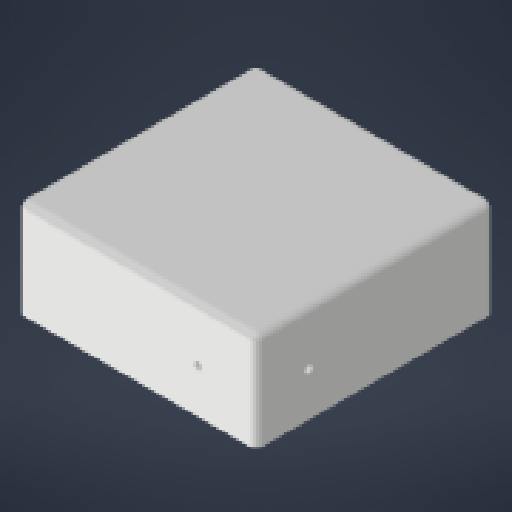
# Autodesk Inventor part: PCB_Housing_02
Saved by Autodesk Inventor 2026.2 (Build 302298000, 298)
## iProperties
Created: 2026-02-05
Part Number: PCB_Housing_02
Material: Generic
Document SubType Name: Modeling
Designer: vckot
Density: 1 g/cm^3
Appearance: Default
Author: vckot
Autodesk Inventor part; units mm, degrees
ref_plane "YZ Plane" through (0, 0, 0) normal (1, 0, 0) x (0, 1, 0)
ref_plane "XZ Plane" through (0, 0, 0) normal (0, 1, 0) x (-1, 0, 0)
ref_plane "XY Plane" through (0, 0, 0) normal (0, 0, 1) x (1, 0, 0)
sketch "Sketch1" plane through (0, 0, 0) normal (0, 1, 0) x (-1, 0, 0)
  line L0 (-85, 85) -> (85, 85)
  line L1 (85, 85) -> (85, -85)
  line L2 (85, -85) -> (-85, -85)
  line L3 (-85, -85) -> (-85, 85)
  line L4 (-85, 85) -> (85, -85) construction
  line L5 (85, 85) -> (-85, -85) construction
  point P0 (0, 0)
  dimension "d0" = 170
  dimension "d1" = 170
  constraints: 12 end point, 2 midpoint, 2 parallel, 1 horizontal, 1 perpendicular
  measures "d0" distance of L0.end L1.end
  measures "d1" distance of L1.end L2.end
extrude "Extrusion1" add sketch "Sketch1" along normal blind 70
fillet "Fillet1" radius 5 8 edges at (0, 70, 85) (85, 70, 0) (-85, 70, 0) (-85, 35, 85) (85, 35, 85) (85, 35, -85) (0, 70, -85) (-85, 35, -85)
shell "Shell1" thickness 4 removed faces 1 at (28.3333, 0, -26.6667)
sketch "Sketch2" plane through (85, 0, 80) normal (1, 0, 0) x (0, 0, -1)
  point P0 (80, 0)
  point P1 (32.5535, 30.9629)
hole "Hole1" at (85, 30.9629, 47.4465) direction (-1, 0, 0) diameter 5 depth 8 tip angle 118
sketch "Sketch3" plane through (-80, 0, 85) normal (0, 0, 1) x (1, 0, 0)
  point P0 (80, 0)
  point P1 (124.013, 31.3444)
hole "Hole2" at (44.013, 31.3444, 85) direction (0, 0, -1) diameter 5 depth 8 tip angle 118
sketch "Sketch4" plane through (-85, 0, -80) normal (-1, 0, 0) x (0, 0, 1)
  point P0 (80, 0)
  point P1 (111.1547, 31.0118)
hole "Hole3" at (-85, 31.0118, 31.1547) direction (1, 0, 0) diameter 5 depth 8 tip angle 118
sketch "Sketch5" plane through (0, 70, 0) normal (0, 1, 0) x (1, 0, 0)
  circle A0 centre (-55.5639, 68.1591) radius 2.5
  circle A1 centre (-49.0639, 68.1591) radius 2.5
  point P0 (0, 0)
  dimension "d27" = 5
  dimension "d28" = 5
  dimension "d29" = 6.5
  constraints: 2 centre point
  measures "d27" diameter of A0
  measures "d28" diameter of A1
  measures "d29" distance of A1.centre A0.centre
extrude "Extrusion2" cut sketch "Sketch5" against normal through all
body "Solid1"
